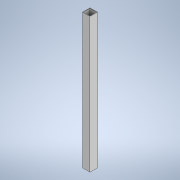
# Autodesk Inventor part: 1x1 Aluminum
Saved by Autodesk Inventor 2020 (Build 240168000, 168)
## iProperties
Created: 2020-01-27
Part Number: 1x1 Aluminum
Material: Generic
Document SubType Name: Modeling
Designer: autum
Density: 1 g/cm^3
Appearance: Default
Author: autum
Autodesk Inventor part; units mm, degrees
ref_plane "YZ Plane" through (0, 0, 0) normal (1, 0, 0) x (0, 1, 0)
ref_plane "XZ Plane" through (0, 0, 0) normal (0, 1, 0) x (-1, 0, 0)
ref_plane "XY Plane" through (0, 0, 0) normal (0, 0, 1) x (1, 0, 0)
sketch "Sketch1" plane through (0, 0, 0) normal (0, 1, 0) x (-1, 0, 0)
  line L0 (-12.7, 12.7) -> (12.7, 12.7)
  line L1 (12.7, 12.7) -> (12.7, -12.7)
  line L2 (12.7, -12.7) -> (-12.7, -12.7)
  line L3 (-12.7, -12.7) -> (-12.7, 12.7)
  line L4 (-12.7, 12.7) -> (12.7, -12.7) construction
  line L5 (12.7, 12.7) -> (-12.7, -12.7) construction
  line L6 (11.1125, 11.1125) -> (-11.1125, 11.1125)
  line L7 (-11.1125, 11.1125) -> (-11.1125, -11.1125)
  line L8 (-11.1125, -11.1125) -> (11.1125, -11.1125)
  line L9 (11.1125, -11.1125) -> (11.1125, 11.1125)
  line L10 (11.1125, 11.1125) -> (-11.1125, -11.1125) construction
  line L11 (-11.1125, 11.1125) -> (11.1125, -11.1125) construction
  point P0 (0, 0)
  dimension "d0" = 25.4
  dimension "d1" = 25.4
  dimension "d2" = 22.225
  dimension "d3" = 22.225
  constraints: 24 end point, 4 midpoint, 4 parallel, 2 horizontal, 2 perpendicular
  measures "d0" distance of L1.end L2.end
  measures "d1" distance of L0.end L1.end
  measures "d2" distance of L8.end L7.end
  measures "d3" distance of L7.end L6.end
extrude "Extrusion1" add sketch "Sketch1" along normal blind 457.2
body "Solid1"
